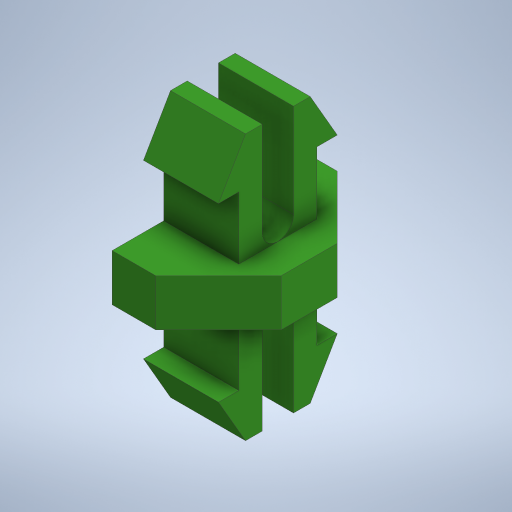
# Autodesk Inventor part: PlugbothWays
Saved by Autodesk Inventor 2024 (Build 280153000, 153)
## iProperties
Created: 2024-01-22
Part Number: PlugbothWays
Material: Generic
Document SubType Name: Modeling
Designer: Admin
Density: 1 g/cm^3
Appearance: Default
Author: Admin
Autodesk Inventor part; units mm, degrees
ref_plane "YZ Plane" through (0, 0, 0) normal (1, 0, 0) x (0, 1, 0)
ref_plane "XZ Plane" through (0, 0, 0) normal (0, 1, 0) x (-1, 0, 0)
ref_plane "XY Plane" through (0, 0, 0) normal (0, 0, 1) x (1, 0, 0)
sketch "Sketch1" plane through (0, 0, 0) normal (0, 1, 0) x (-1, 0, 0)
  line L0 (0, 0) -> (4.8, 0) construction
  line L1 (4.8, 0) -> (4.8, -7.6) construction
  line L2 (4.8, -7.6) -> (0, -7.6) construction
  line L3 (0, -7.6) -> (0, 0) construction
  line L4 (4.8, -9.6) -> (2, -9.6)
  line L5 (2, -9.6) -> (-2, -5.6)
  line L6 (-2, -5.6) -> (-2, -2)
  line L7 (-2, -2) -> (2, 2)
  line L8 (2, 2) -> (4.8, 2)
  line L9 (4.8, 2) -> (4.8, -9.6)
  line L10 (2.4, 0) -> (2.4, 2) construction
  line L11 (-2, -3.8) -> (0, -3.8) construction
  line L12 (2.4, -7.6) -> (2.4, -9.6) construction
  dimension "d0" = 7.6
  dimension "d1" = 4.8
  dimension "d2" = 2
  constraints: 26 end point, 8 midpoint, 6 perpendicular, 3 point on line, 2 equal length, 2 horizontal, 2 parallel
  measures "d0" distance of L0.end L1.end
  measures "d1" distance between parallel lines of L3 L1
  measures "d2" distance between parallel lines of L3 L6
extrude "Extrusion1" add sketch "Sketch1" along normal blind 1.5
sketch "Sketch2" plane through (0, 0, 0) normal (0, -1, 0) x (1, 0, 0)
  line L0 (-4.8, -9.6) -> (-4.8, 2) projected
  line L1 (0, 0) -> (-4.8, 0)
  line L2 (-4.8, 0) -> (-4.8, -7.6)
  line L3 (-4.8, -7.6) -> (0, -7.6)
  line L4 (0, -7.6) -> (0, 0)
  line L5 (2, -5.6) -> (-2, -9.6) projected
  constraints: 8 end point, 2 parallel, 1 horizontal, 1 midpoint, 1 perpendicular, 1 point on line
extrude "Extrusion2" add sketch "Sketch2" along normal blind 7
sketch "Sketch3" plane through (0, 0, 0) normal (1, 0, 0) x (0, 0, -1)
  line L0 (-17.9, 0) -> (-18, 0)
  line L1 (-18, 1) -> (-17.9, 1) construction
  line L2 (0, 0) -> (0, -7)
  line L3 (0, -4) -> (1.7321, -7)
  line L4 (2.8, -7) -> (2.8, 0)
  line L5 (2.8, 0) -> (4.8, 0)
  line L6 (4.8, 0) -> (4.8, -7)
  line L7 (4.8, -7) -> (5.8679, -7)
  line L8 (5.8679, -7) -> (7.6, -4)
  line L9 (7.6, -4) -> (6.3, -4)
  line L10 (6.3, -4) -> (6.3, 0)
  line L11 (7.6, 0) -> (7.6, -7.2498)
  line L12 (6.3, 0) -> (7.6, 0)
  line L13 (2.8, -7) -> (1.7321, -7)
  line L14 (0, -4) -> (1.3, -4)
  line L15 (1.3, -4) -> (1.3, 0)
  line L16 (1.3, 0) -> (0, 0)
  line L17 (0, 0) -> (0, -7)
  line L18 (0, -4) -> (0, -7)
  line L19 (0, -7) -> (1.7321, -7)
  line L20 (7.6, 0) -> (7.6, -4)
  line L21 (3.8, -6.9306) -> (3.8, 0) construction
  line L22 (6.3, -4) -> (4.8, -4) construction
  line L23 (1.3, -4) -> (2.8, -4) construction
  line L24 (-17.9, 0) -> (-18, 0)
  line L25 (-18, 1) -> (-17.9, 1) construction
  line L26 (0, 0) -> (0, -7) projected
  line L27 (2, 0) -> (5.6, 0) projected
  line L28 (7.6, -7) -> (0, -7) projected
  line L29 (2.8, -7) -> (4.8, -7)
  line L30 (5.8679, -7) -> (7.6, -7)
  point P0 (2.8, -7)
  point P1 (4.8, -7)
  dimension "d14" = 4
  dimension "d15" = 1.5
  dimension "d16" = 1
  dimension "d17" = 60
  dimension "d18" = 7.6
  dimension "d20" = 1.3
  constraints: 56 end point, 13 collinear, 6 perpendicular, 5 point on line, 4 vertical, 2 horizontal, 1 midpoint
  measures "d14" distance between parallel lines of L12 L9
  measures "d15" distance between parallel lines of L15 L4
  measures "d16" distance between parallel lines of L21 L6
  measures "d17" angle of L9 L8
  measures "d18" distance between parallel lines of L11 L2
  measures "d20" distance between parallel lines of L11 L10
extrude "Extrusion3" cut sketch "Sketch3" against normal up to surface (4.8 mm away)
fillet "Fillet1" radius 1 2 edges at (-2.4, 0, -4.8) (-2.4, 0, -2.8)
mirror "Mirror1" about plane through (-1.4, 1.5, -3.8) normal (0, 1, 0) of "Extrusion1", "Extrusion2", "Extrusion3", "Fillet1"
body "Solid1"
